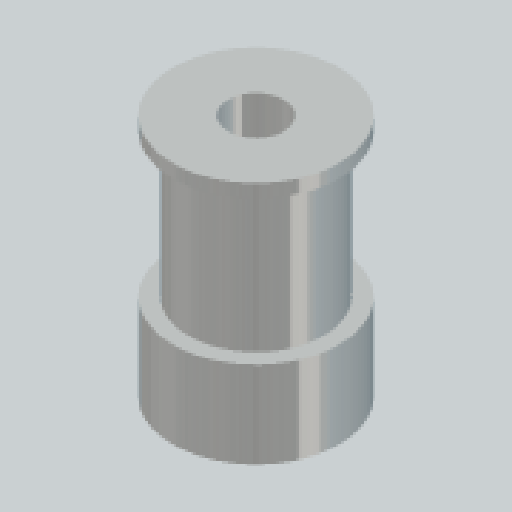
# Autodesk Inventor part: Belt_Pulley_20T
Saved by Autodesk Inventor 2023.2 (Build 272271000, 271)
## iProperties
Created: 2020-05-09
Part Number: Belt_Pulley_20T
Material: Aluminum 6061
Document SubType Name: Modeling
Designer: Remo
Mass: 7.23099 g
Surface Area: 17.0174 cm^2
Volume: 2.67814 cm^3
Density: 2.7 g/cm^3
Appearance: Aluminum - Dark
Description: E3D - Belt Pulley 20 Tooth 12mm
Author: Remo
Autodesk Inventor part; units mm, degrees
ref_plane "YZ Plane" through (0, 0, 0) normal (1, 0, 0) x (0, 1, 0)
ref_plane "XZ Plane" through (0, 0, 0) normal (0, 1, 0) x (-1, 0, 0)
ref_plane "XY Plane" through (0, 0, 0) normal (0, 0, 1) x (1, 0, 0)
sketch "Sketch1" plane through (0, 0, 0) normal (0, 1, 0) x (-1, 0, 0)
  line L0 (0, 0) -> (0, 22)
  line L1 (2.5, 0) -> (2.5, 22)
  line L2 (2.5, 22) -> (7.5, 22)
  line L3 (7.5, 22) -> (7.5, 20.8)
  line L4 (7.5, 20.8) -> (6.1, 20.8)
  line L5 (6.1, 20.8) -> (6.1, 7.8)
  line L6 (6.1, 7.8) -> (7.5, 7.8)
  line L7 (7.5, 7.8) -> (7.5, 0)
  line L8 (7.5, 0) -> (2.5, 0)
  dimension "d0" = 22
  dimension "d1" = 2.5
  dimension "d2" = 7.5
  dimension "d3" = 6.1
  dimension "d4" = 1.2
  dimension "d5" = 7.8
  constraints: 18 end point, 6 perpendicular, 2 horizontal alignment, 2 point on line, 2 vertical
  measures "d0" distance of L0.start L0.end
  measures "d1" distance between parallel lines of L0 L1
  measures "d2" distance between parallel lines of L0 L7
  measures "d3" distance between parallel lines of L0 L5
  measures "d4" distance of L2.end L3.end
  measures "d5" distance of L6.end L7.end
revolve "Revolution1" add sketch "Sketch1" angle 360 about axis through (0, 0, 0) along (0, 0, 1)
body "Solid1"
